Autodesk Inventor part; units mm, degrees
(part 2 of 2)
  line L557 (8.4379, 2.9807) -> (9.3804, 2.9809) construction
  spline S9 degree 3 poles (7.395, 0.9232) (7.395, -0.3765) (7.395, -1.6212) (7.395, -2.8998) (8.7382, -2.8998) (10.0523, -2.8998) (11.3602, -2.8998) (11.3602, -1.608) (11.3602, -0.3479) (11.3602, 0.9232) (10.0298, 0.9232) (8.7267, 0.9232) (7.395, 0.9232) knots 0 0 0 0 1 1 1 2 2 2 3 3 3 4 4 4 4
  line L558 (7.395, 0.9232) -> (7.395, -0.3765) construction
  line L559 (7.395, -0.3765) -> (7.395, -1.6212) construction
  line L560 (7.395, -1.6212) -> (7.395, -2.8998) construction
  line L561 (7.395, -2.8998) -> (8.7382, -2.8998) construction
  line L562 (8.7382, -2.8998) -> (10.0523, -2.8998) construction
  line L563 (10.0523, -2.8998) -> (11.3602, -2.8998) construction
  line L564 (11.3602, -2.8998) -> (11.3602, -1.608) construction
  line L565 (11.3602, -1.608) -> (11.3602, -0.3479) construction
  line L566 (11.3602, -0.3479) -> (11.3602, 0.9232) construction
  line L567 (11.3602, 0.9232) -> (10.0298, 0.9232) construction
  line L568 (10.0298, 0.9232) -> (8.7267, 0.9232) construction
  line L569 (8.7267, 0.9232) -> (7.395, 0.9232) construction
  spline S10 degree 3 poles (13.5547, 21.4139) (13.5547, 20.7978) (13.5547, 20.2145) (13.5547, 19.5876) (13.3856, 19.5794) (13.2295, 19.5656) (13.0735, 19.5654) (11.8356, 19.5635) (10.5968, 19.5355) (9.3599, 19.5716) (7.7939, 19.6173) (7.0047, 18.3535) (7.0798, 17.2739) (7.1726, 15.9402) (8.4636, 14.9664) (9.7967, 15.1936) (10.723, 15.3515) (11.7606, 15.9826) (11.6553, 17.3708) (11.6155, 17.896) (11.6488, 18.4267) (11.6488, 18.9818) (12.2921, 18.9818) (12.9033, 18.9818) (13.5455, 18.9818) (13.5455, 17.0836) (13.5455, 15.191) (13.5455, 13.2651) (10.7965, 13.2651) (8.0517, 13.2651) (5.2802, 13.2651) (5.2802, 15.9827) (5.2802, 18.6862) (5.2802, 21.4139) (8.0328, 21.4139) (10.7687, 21.4139) (13.5547, 21.4139) knots 0 0 0 0 1 1 1 2 2 2 3 3 3 4 4 4 5 5 5 6 6 6 7 7 7 8 8 8 9 9 9 10 10 10 11 11 11 12 12 12 12
  line L570 (13.5547, 21.4139) -> (13.5547, 20.7978) construction
  line L571 (13.5547, 20.7978) -> (13.5547, 20.2145) construction
  line L572 (13.5547, 20.2145) -> (13.5547, 19.5876) construction
  line L573 (13.5547, 19.5876) -> (13.3856, 19.5794) construction
  line L574 (13.3856, 19.5794) -> (13.2295, 19.5656) construction
  line L575 (13.2295, 19.5656) -> (13.0735, 19.5654) construction
  line L576 (13.0735, 19.5654) -> (11.8356, 19.5635) construction
  line L577 (11.8356, 19.5635) -> (10.5968, 19.5355) construction
  line L578 (10.5968, 19.5355) -> (9.3599, 19.5716) construction
  line L579 (9.3599, 19.5716) -> (7.7939, 19.6173) construction
  line L580 (7.7939, 19.6173) -> (7.0047, 18.3535) construction
  line L581 (7.0047, 18.3535) -> (7.0798, 17.2739) construction
  line L582 (7.0798, 17.2739) -> (7.1726, 15.9402) construction
  line L583 (7.1726, 15.9402) -> (8.4636, 14.9664) construction
  line L584 (8.4636, 14.9664) -> (9.7967, 15.1936) construction
  line L585 (9.7967, 15.1936) -> (10.723, 15.3515) construction
  line L586 (10.723, 15.3515) -> (11.7606, 15.9826) construction
  line L587 (11.7606, 15.9826) -> (11.6553, 17.3708) construction
  line L588 (11.6553, 17.3708) -> (11.6155, 17.896) construction
  line L589 (11.6155, 17.896) -> (11.6488, 18.4267) construction
  line L590 (11.6488, 18.4267) -> (11.6488, 18.9818) construction
  line L591 (11.6488, 18.9818) -> (12.2921, 18.9818) construction
  line L592 (12.2921, 18.9818) -> (12.9033, 18.9818) construction
  line L593 (12.9033, 18.9818) -> (13.5455, 18.9818) construction
  line L594 (13.5455, 18.9818) -> (13.5455, 17.0836) construction
  line L595 (13.5455, 17.0836) -> (13.5455, 15.191) construction
  line L596 (13.5455, 15.191) -> (13.5455, 13.2651) construction
  line L597 (13.5455, 13.2651) -> (10.7965, 13.2651) construction
  line L598 (10.7965, 13.2651) -> (8.0517, 13.2651) construction
  line L599 (8.0517, 13.2651) -> (5.2802, 13.2651) construction
  line L600 (5.2802, 13.2651) -> (5.2802, 15.9827) construction
  line L601 (5.2802, 15.9827) -> (5.2802, 18.6862) construction
  line L602 (5.2802, 18.6862) -> (5.2802, 21.4139) construction
  line L603 (5.2802, 21.4139) -> (8.0328, 21.4139) construction
  line L604 (8.0328, 21.4139) -> (10.7687, 21.4139) construction
  line L605 (10.7687, 21.4139) -> (13.5547, 21.4139) construction
  spline S11 degree 3 poles (12.3909, 18.3321) (12.3909, 17.9593) (12.3924, 17.6224) (12.3907, 17.2856) (12.3829, 15.79) (11.3598, 14.6634) (9.8286, 14.4632) (8.263, 14.2585) (6.9991, 15.046) (6.5727, 16.4766) (6.0175, 18.3392) (7.3361, 20.3592) (9.3492, 20.2235) (9.9068, 20.1859) (10.4692, 20.2178) (11.0293, 20.2178) (11.6291, 20.2178) (12.2288, 20.2178) (12.8345, 20.2178) (12.8345, 20.422) (12.8345, 20.5718) (12.8345, 20.7162) (10.5052, 20.7162) (8.2116, 20.7162) (5.9125, 20.7162) (5.9125, 18.4444) (5.9125, 16.1995) (5.9125, 13.9485) (8.2378, 13.9485) (10.5306, 13.9485) (12.8399, 13.9485) (12.8399, 15.4213) (12.8399, 16.8701) (12.8399, 18.3321) (12.6931, 18.3321) (12.5778, 18.3321) (12.3909, 18.3321) knots 0 0 0 0 1 1 1 2 2 2 3 3 3 4 4 4 5 5 5 6 6 6 7 7 7 8 8 8 9 9 9 10 10 10 11 11 11 12 12 12 12
  line L606 (12.3909, 18.3321) -> (12.3909, 17.9593) construction
  line L607 (12.3909, 17.9593) -> (12.3924, 17.6224) construction
  line L608 (12.3924, 17.6224) -> (12.3907, 17.2856) construction
  line L609 (12.3907, 17.2856) -> (12.3829, 15.79) construction
  line L610 (12.3829, 15.79) -> (11.3598, 14.6634) construction
  line L611 (11.3598, 14.6634) -> (9.8286, 14.4632) construction
  line L612 (9.8286, 14.4632) -> (8.263, 14.2585) construction
  line L613 (8.263, 14.2585) -> (6.9991, 15.046) construction
  line L614 (6.9991, 15.046) -> (6.5727, 16.4766) construction
  line L615 (6.5727, 16.4766) -> (6.0175, 18.3392) construction
  line L616 (6.0175, 18.3392) -> (7.3361, 20.3592) construction
  line L617 (7.3361, 20.3592) -> (9.3492, 20.2235) construction
  line L618 (9.3492, 20.2235) -> (9.9068, 20.1859) construction
  line L619 (9.9068, 20.1859) -> (10.4692, 20.2178) construction
  line L620 (10.4692, 20.2178) -> (11.0293, 20.2178) construction
  line L621 (11.0293, 20.2178) -> (11.6291, 20.2178) construction
  line L622 (11.6291, 20.2178) -> (12.2288, 20.2178) construction
  line L623 (12.2288, 20.2178) -> (12.8345, 20.2178) construction
  line L624 (12.8345, 20.2178) -> (12.8345, 20.422) construction
  line L625 (12.8345, 20.422) -> (12.8345, 20.5718) construction
  line L626 (12.8345, 20.5718) -> (12.8345, 20.7162) construction
  line L627 (12.8345, 20.7162) -> (10.5052, 20.7162) construction
  line L628 (10.5052, 20.7162) -> (8.2116, 20.7162) construction
  line L629 (8.2116, 20.7162) -> (5.9125, 20.7162) construction
  line L630 (5.9125, 20.7162) -> (5.9125, 18.4444) construction
  line L631 (5.9125, 18.4444) -> (5.9125, 16.1995) construction
  line L632 (5.9125, 16.1995) -> (5.9125, 13.9485) construction
  line L633 (5.9125, 13.9485) -> (8.2378, 13.9485) construction
  line L634 (8.2378, 13.9485) -> (10.5306, 13.9485) construction
  line L635 (10.5306, 13.9485) -> (12.8399, 13.9485) construction
  line L636 (12.8399, 13.9485) -> (12.8399, 15.4213) construction
  line L637 (12.8399, 15.4213) -> (12.8399, 16.8701) construction
  line L638 (12.8399, 16.8701) -> (12.8399, 18.3321) construction
  line L639 (12.8399, 18.3321) -> (12.6931, 18.3321) construction
  line L640 (12.6931, 18.3321) -> (12.5778, 18.3321) construction
  line L641 (12.5778, 18.3321) -> (12.3909, 18.3321) construction
  spline S12 degree 3 poles (7.395, 0.9232) (8.7267, 0.9232) (10.0298, 0.9232) (11.3602, 0.9232) (11.3602, -0.3479) (11.3602, -1.608) (11.3602, -2.8998) (10.0523, -2.8998) (8.7382, -2.8998) (7.395, -2.8998) (7.395, -1.6212) (7.395, -0.3765) (7.395, 0.9232) knots 0 0 0 0 1 1 1 2 2 2 3 3 3 4 4 4 4
  line L642 (7.395, 0.9232) -> (8.7267, 0.9232) construction
  line L643 (8.7267, 0.9232) -> (10.0298, 0.9232) construction
  line L644 (10.0298, 0.9232) -> (11.3602, 0.9232) construction
  line L645 (11.3602, 0.9232) -> (11.3602, -0.3479) construction
  line L646 (11.3602, -0.3479) -> (11.3602, -1.608) construction
  line L647 (11.3602, -1.608) -> (11.3602, -2.8998) construction
  line L648 (11.3602, -2.8998) -> (10.0523, -2.8998) construction
  line L649 (10.0523, -2.8998) -> (8.7382, -2.8998) construction
  line L650 (8.7382, -2.8998) -> (7.395, -2.8998) construction
  line L651 (7.395, -2.8998) -> (7.395, -1.6212) construction
  line L652 (7.395, -1.6212) -> (7.395, -0.3765) construction
  line L653 (7.395, -0.3765) -> (7.395, 0.9232) construction
  spline S13 degree 3 poles (12.3909, 18.3321) (12.5778, 18.3321) (12.6931, 18.3321) (12.8399, 18.3321) (12.8399, 16.8701) (12.8399, 15.4213) (12.8399, 13.9485) (10.5306, 13.9485) (8.2378, 13.9485) (5.9125, 13.9485) (5.9125, 16.1995) (5.9125, 18.4444) (5.9125, 20.7162) (8.2116, 20.7162) (10.5052, 20.7162) (12.8345, 20.7162) (12.8345, 20.5718) (12.8345, 20.422) (12.8345, 20.2178) (12.2288, 20.2178) (11.6291, 20.2178) (11.0293, 20.2178) (10.4692, 20.2178) (9.9068, 20.1859) (9.3492, 20.2235) (7.3361, 20.3592) (6.0175, 18.3392) (6.5727, 16.4766) (6.9991, 15.046) (8.263, 14.2585) (9.8286, 14.4632) (11.3598, 14.6634) (12.3829, 15.79) (12.3907, 17.2856) (12.3924, 17.6224) (12.3909, 17.9593) (12.3909, 18.3321) knots 0 0 0 0 1 1 1 2 2 2 3 3 3 4 4 4 5 5 5 6 6 6 7 7 7 8 8 8 9 9 9 10 10 10 11 11 11 12 12 12 12
  line L654 (12.3909, 18.3321) -> (12.5778, 18.3321) construction
  line L655 (12.5778, 18.3321) -> (12.6931, 18.3321) construction
  line L656 (12.6931, 18.3321) -> (12.8399, 18.3321) construction
  line L657 (12.8399, 18.3321) -> (12.8399, 16.8701) construction
  line L658 (12.8399, 16.8701) -> (12.8399, 15.4213) construction
  line L659 (12.8399, 15.4213) -> (12.8399, 13.9485) construction
  line L660 (12.8399, 13.9485) -> (10.5306, 13.9485) construction
  line L661 (10.5306, 13.9485) -> (8.2378, 13.9485) construction
  line L662 (8.2378, 13.9485) -> (5.9125, 13.9485) construction
  line L663 (5.9125, 13.9485) -> (5.9125, 16.1995) construction
  line L664 (5.9125, 16.1995) -> (5.9125, 18.4444) construction
  line L665 (5.9125, 18.4444) -> (5.9125, 20.7162) construction
  line L666 (5.9125, 20.7162) -> (8.2116, 20.7162) construction
  line L667 (8.2116, 20.7162) -> (10.5052, 20.7162) construction
  line L668 (10.5052, 20.7162) -> (12.8345, 20.7162) construction
  line L669 (12.8345, 20.7162) -> (12.8345, 20.5718) construction
  line L670 (12.8345, 20.5718) -> (12.8345, 20.422) construction
  line L671 (12.8345, 20.422) -> (12.8345, 20.2178) construction
  line L672 (12.8345, 20.2178) -> (12.2288, 20.2178) construction
  line L673 (12.2288, 20.2178) -> (11.6291, 20.2178) construction
  line L674 (11.6291, 20.2178) -> (11.0293, 20.2178) construction
  line L675 (11.0293, 20.2178) -> (10.4692, 20.2178) construction
  line L676 (10.4692, 20.2178) -> (9.9068, 20.1859) construction
  line L677 (9.9068, 20.1859) -> (9.3492, 20.2235) construction
  line L678 (9.3492, 20.2235) -> (7.3361, 20.3592) construction
  line L679 (7.3361, 20.3592) -> (6.0175, 18.3392) construction
  line L680 (6.0175, 18.3392) -> (6.5727, 16.4766) construction
  line L681 (6.5727, 16.4766) -> (6.9991, 15.046) construction
  line L682 (6.9991, 15.046) -> (8.263, 14.2585) construction
  line L683 (8.263, 14.2585) -> (9.8286, 14.4632) construction
  line L684 (9.8286, 14.4632) -> (11.3598, 14.6634) construction
  line L685 (11.3598, 14.6634) -> (12.3829, 15.79) construction
  line L686 (12.3829, 15.79) -> (12.3907, 17.2856) construction
  line L687 (12.3907, 17.2856) -> (12.3924, 17.6224) construction
  line L688 (12.3924, 17.6224) -> (12.3909, 17.9593) construction
  line L689 (12.3909, 17.9593) -> (12.3909, 18.3321) construction
  point P0 (0, 0)
  constraints: 22 other
extrude "Extrusion2" add sketch "Sketch2" along normal blind 0.635
equation "\"d2\" = 0.5 * d0"
equation "\"d3\" = 0.5 * d1"
body "Solid1"
